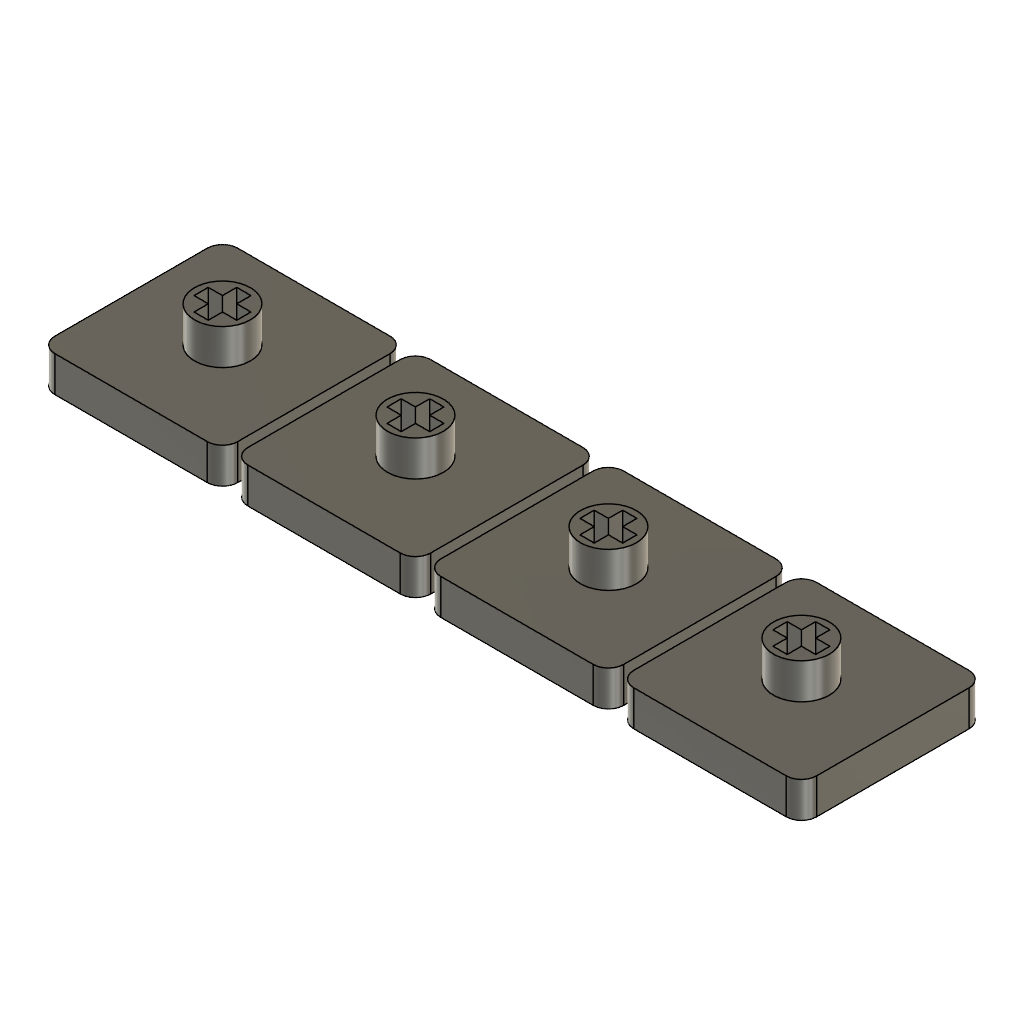
capuchons (Autodesk Fusion 360 design; units mm, degrees)
part number: 2026-09-27-10-10-05-770
Autodesk Fusion 360 part; units mm, degrees
sketch "Esquisse14" plane through (0, 0, 0) normal (0, 0, 1) x (1, 0, 0)
  line L0 (9, 9) -> (-9, 9)
  line L1 (-9, 9) -> (-9, -9)
  line L2 (-9, -9) -> (9, -9)
  line L3 (9, -9) -> (9, 9)
  line L4 (9, 9) -> (-9, -9) construction
  line L5 (-9, 9) -> (9, -9) construction
  dimension "d78" = 18
  dimension "d79" = 18
  constraint horizontal L0
  constraint perpendicular L0 L1
  constraint parallel L0 L2
  constraint parallel L1 L3
  constraint coincident L4 origin
  constraint coincident L5 origin
  measures "d78" distance of L0.end L1.end
  measures "d79" distance of L0.start L0.end
extrude "Extrusion14" add sketch "Esquisse14" along normal blind 3.5 makes body 1
fillet "Congé9" radius 1.5 4 edges at (-9, -9, 1.75) (9, -9, 1.75) (9, 9, 1.75) (-9, 9, 1.75) on bodies 1
sketch "Esquisse15" plane through (0, 0, 3.5) normal (0, 0, 1) x (-1, 0, 0)
  arc A0 (7.5, -9) -> (9, -7.5) centre (7.5, -7.5) ccw
  line L0 (9, -7.5) -> (9, 7.5)
  arc A1 (9, 7.5) -> (7.5, 9) centre (7.5, 7.5) ccw
  line L1 (7.5, 9) -> (-7.5, 9)
  arc A2 (-7.5, 9) -> (-9, 7.5) centre (-7.5, 7.5) ccw
  line L2 (-9, 7.5) -> (-9, -7.5)
  arc A3 (-9, -7.5) -> (-7.5, -9) centre (-7.5, -7.5) ccw
  line L3 (-7.5, -9) -> (7.5, -9)
  circle A4 centre (0, 0) radius 2.75
  dimension "d84" = 5.5
  constraint coincident A4.centre origin
  measures "d84" diameter of A4
extrude "Extrusion15" add sketch "Esquisse15" along normal blind 3.5 separate body contours A4 makes body 2
sketch "Esquisse16" plane through (0, 0, 7) normal (0, 0, 1) x (-1, 0, 0)
  circle A0 centre (0, 0) radius 2.75
  line L0 (2.1, -0.7) -> (-2.1, -0.7)
  line L1 (-2.1, -0.7) -> (-2.1, 0.7)
  line L2 (-2.1, 0.7) -> (2.1, 0.7)
  line L3 (2.1, 0.7) -> (2.1, -0.7)
  line L4 (2.1, -0.7) -> (-2.1, 0.7) construction
  line L5 (-2.1, -0.7) -> (2.1, 0.7) construction
  dimension "d87" = 4.2
  dimension "d88" = 1.4
  constraint horizontal L0
  constraint perpendicular L0 L1
  constraint parallel L0 L2
  constraint parallel L1 L3
  constraint coincident L4 A0.centre
  constraint coincident L5 A0.centre
  constraint coincident A0.centre origin
  measures "d87" distance of L1.end L2.end
  measures "d88" distance of L0.end L1.end
extrude "Extrusion16" cut sketch "Esquisse16" against normal blind 3.5 contours L0 L1 L2 L3 bodies 2
sketch "Esquisse17" plane through (0, 0, 7) normal (0, 0, 1) x (-1, 0, 0)
  line L0 (-2.1, -0.7) -> (-2.1, 0.7)
  line L1 (-2.1, 0.7) -> (2.1, 0.7)
  line L2 (2.1, 0.7) -> (2.1, -0.7)
  line L3 (2.1, -0.7) -> (-2.1, -0.7)
  circle A0 centre (0, 0) radius 2.75
  line L4 (0.7, -2.1) -> (-0.7, -2.1)
  line L5 (-0.7, -2.1) -> (-0.7, 2.1)
  line L6 (-0.7, 2.1) -> (0.7, 2.1)
  line L7 (0.7, 2.1) -> (0.7, -2.1)
  line L8 (0.7, -2.1) -> (-0.7, 2.1) construction
  line L9 (-0.7, -2.1) -> (0.7, 2.1) construction
  dimension "d91" = 1.4
  dimension "d92" = 4.2
  constraint horizontal L4
  constraint perpendicular L4 L5
  constraint parallel L4 L6
  constraint parallel L5 L7
  constraint coincident L8 A0.centre
  constraint coincident L9 A0.centre
  constraint coincident A0.centre origin
  measures "d91" distance of L5.end L6.end
  measures "d92" distance of L4.start L6.end
extrude "Extrusion17" cut sketch "Esquisse17" against normal blind 3.5 contours L3 L4 L5 L7 | L1 L5 L6 L7 bodies 2
sketch "Esquisse18" plane through (0, 0, 0) normal (0, 0, 1) x (1, 0, 0)
  line L0 (-0.4, -2.5) -> (0.4, -2.5)
  line L1 (0.4, -2.5) -> (0.4, 2.5)
  line L2 (0.4, 2.5) -> (-0.4, 2.5)
  line L3 (-0.4, 2.5) -> (-0.4, -2.5)
  line L4 (-0.4, -2.5) -> (0.4, 2.5) construction
  line L5 (0.4, -2.5) -> (-0.4, 2.5) construction
  dimension "d95" = 0.8
  dimension "d96" = 5
  constraint horizontal L0
  constraint perpendicular L0 L1
  constraint parallel L0 L2
  constraint parallel L1 L3
  constraint coincident L4 origin
  constraint coincident L5 origin
  measures "d95" distance of L1.end L2.end
  measures "d96" distance of L0.end L1.end
combine "Combiner1" operation add target body 1 tool bodies 2
pattern_linear "Réseau R1" count 4 spacing 19 along (1, 0, 0) of bodies 1 makes body 3 at (16, 2.5, 0) makes body 4 at (35.5, -2, 0) makes body 5 at (60, -2.5, 0)
extrude "Extrusion18" cut sketch "Esquisse18" along normal blind 0.6 bodies 1
sketch "Esquisse19" plane through (0, 0, 0) normal (0, 0, 1) x (1, 0, 0)
  line L0 (-0.4, 2.5) -> (0.4, 2.5)
  line L1 (0.4, 2.5) -> (0.4, -2.5)
  line L2 (0.4, -2.5) -> (-0.4, -2.5)
  line L3 (-0.4, -2.5) -> (-0.4, 2.5)
  line L4 (-0.4, 2.5) -> (0.4, -2.5) construction
  line L5 (0.4, 2.5) -> (-0.4, -2.5) construction
  line L6 (1.1, 2.5) -> (1.9, 2.5)
  line L7 (1.9, 2.5) -> (1.9, -2.5)
  line L8 (1.9, -2.5) -> (1.1, -2.5)
  line L9 (1.1, -2.5) -> (1.1, 2.5)
  line L10 (1.1, 2.5) -> (1.9, -2.5) construction
  line L11 (1.9, 2.5) -> (1.1, -2.5) construction
  point P0 (1.5, 0)
  dimension "d99" = 0.8
  dimension "d100" = 5
  dimension "d101" = 0.8
  dimension "d102" = 5
  dimension "d103" = 1.5
  constraint horizontal L0
  constraint perpendicular L0 L1
  constraint parallel L0 L2
  constraint parallel L1 L3
  constraint coincident L4 origin
  constraint coincident L5 origin
  constraint horizontal L6
  constraint perpendicular L6 L7
  constraint parallel L6 L8
  constraint parallel L7 L9
  constraint coincident L10 P0
  constraint coincident L11 P0
  measures "d99" distance of L1.end L2.end
  measures "d100" distance of L0.end L1.end
  measures "d101" distance of L6.start L6.end
  measures "d102" distance of L6.end L7.end
  measures "d103" distance of origin P0
extrude "Extrusion19" cut sketch "Esquisse19" along normal blind 0.6 contours L6 L7 L8 L9 bodies 1
sketch "Esquisse20" plane through (0, 0, 0) normal (0, 0, 1) x (1, 0, 0)
  line L0 (-1.9, -2.5) -> (-1.1, -2.5)
  line L1 (-1.1, -2.5) -> (-1.1, 2.5)
  line L2 (-1.1, 2.5) -> (-1.9, 2.5)
  line L3 (-1.9, 2.5) -> (-1.9, -2.5)
  line L4 (-1.9, -2.5) -> (-1.1, 2.5) construction
  line L5 (-1.1, -2.5) -> (-1.9, 2.5) construction
  point P0 (-1.5, 0)
  dimension "d106" = 5
  dimension "d107" = 0.8
  dimension "d108" = 1.5
  constraint horizontal L0
  constraint perpendicular L0 L1
  constraint parallel L0 L2
  constraint parallel L1 L3
  constraint coincident L4 P0
  constraint coincident L5 P0
  measures "d106" distance of L0.start L2.end
  measures "d107" distance of L1.end L2.end
  measures "d108" distance of origin P0
extrude "Extrusion20" cut sketch "Esquisse20" along normal blind 0.6 bodies 1
sketch "Esquisse13" plane through (0, 0, 6.5) normal (0, 0, 1) x (-1, 0, 0)
  line L0 (2.1, 0.7) -> (2.1, -0.7)
  line L1 (2.1, -0.7) -> (-2.1, -0.7)
  line L2 (-2.1, -0.7) -> (-2.1, 0.7)
  line L3 (-2.1, 0.7) -> (2.1, 0.7)
  circle A0 centre (0, 0) radius 2.75
  line L4 (-0.7, 2.1) -> (0.7, 2.1)
  line L5 (0.7, 2.1) -> (0.7, -2.1)
  line L6 (0.7, -2.1) -> (-0.7, -2.1)
  line L7 (-0.7, -2.1) -> (-0.7, 2.1)
  line L8 (-0.7, 2.1) -> (0.7, -2.1) construction
  line L9 (0.7, 2.1) -> (-0.7, -2.1) construction
  dimension "d74" = 1.4
  dimension "d75" = 4.2
  constraint horizontal L4
  constraint perpendicular L4 L5
  constraint parallel L4 L6
  constraint parallel L5 L7
  constraint coincident L8 A0.centre
  constraint coincident L9 A0.centre
  constraint coincident A0.centre origin
  measures "d74" distance of L5.end L6.end
  measures "d75" distance of L4.start L6.end
sketch "Esquisse21" plane through (0, 0, 0) normal (0, 0, -1) x (1, 0, 0)
  arc A0 (10, -7.5) -> (11.5, -9) centre (11.5, -7.5) ccw
  line L0 (11.5, -9) -> (26.5, -9)
  arc A1 (26.5, -9) -> (28, -7.5) centre (26.5, -7.5) ccw
  line L1 (28, -7.5) -> (28, 7.5)
  arc A2 (28, 7.5) -> (26.5, 9) centre (26.5, 7.5) ccw
  line L2 (26.5, 9) -> (11.5, 9)
  arc A3 (11.5, 9) -> (10, 7.5) centre (11.5, 7.5) ccw
  line L3 (10, 7.5) -> (10, -7.5)
  line L4 (19.4, -2.5) -> (18.6, -2.5)
  line L5 (18.6, -2.5) -> (18.6, 2.5)
  line L6 (18.6, 2.5) -> (19.4, 2.5)
  line L7 (19.4, 2.5) -> (19.4, -2.5)
  line L8 (19.4, -2.5) -> (18.6, 2.5) construction
  line L9 (18.6, -2.5) -> (19.4, 2.5) construction
  point P0 (19, 0)
  dimension "d115" = 0.8
  dimension "d116" = 5
  constraint horizontal L4
  constraint perpendicular L4 L5
  constraint parallel L4 L6
  constraint parallel L5 L7
  constraint coincident L8 P0
  constraint coincident L9 P0
  measures "d115" distance of L5.end L6.end
  measures "d116" distance of L4.end L5.end
extrude "Extrusion21" cut sketch "Esquisse21" against normal blind 0.6 contours L4 L5 L6 L7 bodies 3
sketch "Esquisse22" plane through (0, 0, 0) normal (0, 0, -1) x (1, 0, 0)
  arc A0 (29, -7.5) -> (30.5, -9) centre (30.5, -7.5) ccw
  line L0 (30.5, -9) -> (45.5, -9)
  arc A1 (45.5, -9) -> (47, -7.5) centre (45.5, -7.5) ccw
  line L1 (47, -7.5) -> (47, 7.5)
  arc A2 (47, 7.5) -> (45.5, 9) centre (45.5, 7.5) ccw
  line L2 (45.5, 9) -> (30.5, 9)
  arc A3 (30.5, 9) -> (29, 7.5) centre (30.5, 7.5) ccw
  line L3 (29, 7.5) -> (29, -7.5)
  line L4 (37.9, -2.5452) -> (37.1, -2.5452)
  line L5 (37.1, -2.5452) -> (37.1, 2.4548)
  line L6 (37.1, 2.4548) -> (37.9, 2.4548)
  line L7 (37.9, 2.4548) -> (37.9, -2.5452)
  line L8 (37.9, -2.5452) -> (37.1, 2.4548) construction
  line L9 (37.1, -2.5452) -> (37.9, 2.4548) construction
  point P0 (37.5, -0.0452)
  dimension "d119" = 0.8
  dimension "d120" = 5
  constraint horizontal L4
  constraint perpendicular L4 L5
  constraint parallel L4 L6
  constraint parallel L5 L7
  constraint coincident L8 P0
  constraint coincident L9 P0
  measures "d119" distance of L5.end L6.end
  measures "d120" distance of L4.end L5.end
extrude "Extrusion22" cut sketch "Esquisse22" against normal blind 0.6 contours L4 L5 L6 L7 bodies 4
sketch "Esquisse23" plane through (0, 0, 0) normal (0, 0, -1) x (1, 0, 0)
  line L0 (37.1, -2.5452) -> (37.1, 2.4548)
  line L1 (37.1, 2.4548) -> (37.9, 2.4548)
  line L2 (37.9, 2.4548) -> (37.9, -2.5452)
  line L3 (37.9, -2.5452) -> (37.1, -2.5452)
  arc A0 (29, -7.5) -> (30.5, -9) centre (30.5, -7.5) ccw
  line L4 (30.5, -9) -> (45.5, -9)
  arc A1 (45.5, -9) -> (47, -7.5) centre (45.5, -7.5) ccw
  line L5 (47, -7.5) -> (47, 7.5)
  arc A2 (47, 7.5) -> (45.5, 9) centre (45.5, 7.5) ccw
  line L6 (45.5, 9) -> (30.5, 9)
  arc A3 (30.5, 9) -> (29, 7.5) centre (30.5, 7.5) ccw
  line L7 (29, 7.5) -> (29, -7.5)
  line L8 (39.3012, -2.5452) -> (38.5012, -2.5452)
  line L9 (38.5012, -2.5452) -> (38.5012, 2.4548)
  line L10 (38.5012, 2.4548) -> (39.3012, 2.4548)
  line L11 (39.3012, 2.4548) -> (39.3012, -2.5452)
  line L12 (39.3012, -2.5452) -> (38.5012, 2.4548) construction
  line L13 (38.5012, -2.5452) -> (39.3012, 2.4548) construction
  point P0 (38.9012, -0.0452)
  dimension "d123" = 5
  dimension "d124" = 0.8
  constraint horizontal L8
  constraint perpendicular L8 L9
  constraint parallel L8 L10
  constraint parallel L9 L11
  constraint coincident L12 P0
  constraint coincident L13 P0
  measures "d123" distance of L8.start L10.end
  measures "d124" distance of L9.end L10.end
extrude "Extrusion23" cut sketch "Esquisse23" against normal blind 0.6 contours L8 L9 L10 L11 bodies 4
sketch "Esquisse25" plane through (0, 0, 0) normal (0, 0, -1) x (1, 0, 0)
  arc A0 (48, -7.5) -> (49.5, -9) centre (49.5, -7.5) ccw
  line L0 (49.5, -9) -> (64.5, -9)
  arc A1 (64.5, -9) -> (66, -7.5) centre (64.5, -7.5) ccw
  line L1 (66, -7.5) -> (66, 7.5)
  arc A2 (66, 7.5) -> (64.5, 9) centre (64.5, 7.5) ccw
  line L2 (64.5, 9) -> (49.5, 9)
  arc A3 (49.5, 9) -> (48, 7.5) centre (49.5, 7.5) ccw
  line L3 (48, 7.5) -> (48, -7.5)
  circle A4 centre (57, 0) radius 2.5
  dimension "d129" = 5
  measures "d129" diameter of A4
extrude "Extrusion24" cut sketch "Esquisse25" against normal blind 0.6 contours A4 bodies 5
equation "cote = 35 mm"
equation "largeur = 30 mm"
equation "epaisseur = 4 mm"
equation "p_aiment = 2.2 mm"
equation "d_aimant = 6.2 mm"
